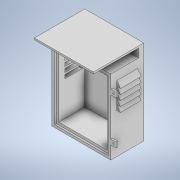
# Autodesk Inventor part: Part6
Saved by Autodesk Inventor 2022.6 (Build 266554010, 554A)
## iProperties
Created: 2025-03-19
Part Number: Part6
Material: Generic
Document SubType Name: Modeling
Designer: khinm
Density: 1 g/cm^3
Appearance: Default
Author: khinm
Autodesk Inventor part; units mm, degrees
sketch "Sketch2" plane through (0, 0, 0) normal (1, 0, 0) x (0, 1, 0)
  line L0 (215, 47.5) -> (0, 47.5)
  line L1 (0, 47.5) -> (0, -47.5)
  line L2 (0, -47.5) -> (215, -47.5)
  line L3 (215, -47.5) -> (215, 47.5)
  point P0 (0, 0)
  point P1 (0, 0)
  dimension "d0" = 95
  dimension "d1" = 215
  constraints: 8 end point, 2 parallel, 1 coincident, 1 horizontal, 1 midpoint, 1 perpendicular
  measures "d0" distance of L2.end L0.start
  measures "d1" distance from line of L1.end L3
extrude "Extrusion1" add sketch "Sketch2" along normal mid plane 170
sketch "Sketch3" plane through (-85, 0, 47.5) normal (0, 0, 1) x (1, 0, 0)
  line L0 (15, 200) -> (155, 200)
  line L1 (155, 200) -> (155, 15)
  line L2 (155, 15) -> (15, 15)
  line L3 (15, 15) -> (15, 200)
  line L4 (170, 0) -> (0, 0) projected
  line L5 (0, 215) -> (170, 215) projected
  line L6 (0, 0) -> (0, 215) projected
  line L7 (170, 215) -> (170, 0) projected
  point P0 (85, 0)
  point P1 (85, 0)
  point P2 (85, 15)
  dimension "d4" = 15
  dimension "d5" = 15
  dimension "d6" = 15
  dimension "d7" = 15
  constraints: 8 end point, 2 midpoint, 2 parallel, 1 horizontal, 1 perpendicular, 1 vertical alignment
  measures "d4" distance between parallel lines of L5 L0
  measures "d5" distance between parallel lines of L4 L2
  measures "d6" distance between parallel lines of L6 L3
  measures "d7" distance between parallel lines of L1 L7
extrude "Extrusion2" cut sketch "Sketch3" against normal blind 80 contours L0 L1 L2 L3
ref_plane "Work Plane1" through (0, 0, 0) normal (1, 0, 0) x (0, 1, 0)
sketch "Sketch4" plane through (0, 0, 0) normal (1, 0, 0) x (0, 1, 0)
  line L0 (200, 47.5) -> (200, -32.5) projected
  line L1 (15, 47.5) -> (200, 47.5) projected
  line L2 (200, 47.5) -> (207.5, 47.5)
  line L3 (207.5, 47.5) -> (207.5, 42.5)
  line L4 (207.5, 42.5) -> (200, 42.5)
  line L5 (200, 42.5) -> (200, 47.5)
  point P0 (0, 0)
  point P1 (200, 45)
  point P2 (207.5, 45)
  point P3 (203.75, 42.5)
  point P4 (203.75, 47.5)
  dimension "d12" = 7.5
  dimension "d13" = 5
  constraints: 8 end point, 4 midpoint, 2 parallel, 1 horizontal, 1 perpendicular
  measures "d12" distance of point (200, 45) point (207.5, 45)
  measures "d13" distance of point (203.75, 42.5) point (203.75, 47.5)
sketch3d "3D Sketch1"
  line L0 (-70, 200, 47.5) -> (-70, 15, 47.5)
  line L1 (-70, 15, 47.5) -> (70, 15, 47.5)
  line L2 (70, 15, 47.5) -> (70, 200, 47.5)
  line L3 (70, 200, 47.5) -> (-70, 200, 47.5)
sweep "Sweep1" cut profiles "Sketch4" path "3D Sketch1"
ref_plane "Work Plane2" through (0, 0, 0) normal (0, 0, 1) x (1, 0, 0)
sketch "Sketch6" plane through (0, 0, 0) normal (0, 0, 1) x (1, 0, 0)
  line L0 (85, 0) -> (85, 215) projected
  line L1 (85, 190) -> (85, 175)
  line L2 (85, 175) -> (95, 175)
  line L3 (95, 175) -> (85, 190)
  point P0 (0, 0)
  dimension "d17" = 25
  dimension "d18" = 15
  dimension "d19" = 10
  dimension "d23" = 56.31
  constraints: 6 end point, 2 point on line, 1 horizontal
  measures "d17" distance of L1.start L0.end
  measures "d18" distance of L1.end L1.start
  measures "d19" distance of L1.end L2.end
  measures "d23" angle of L3 L2
extrude "Extrusion3" add sketch "Sketch6" along normal mid plane 60
sketch "Sketch7" plane through (0, 0, 0) normal (0, 0, 1) x (1, 0, 0)
  line L0 (70, 200) -> (70, 15) projected
  line L1 (70, 175) -> (91.6667, 175)
  line L2 (85, 0) -> (85, 215) projected
  line L3 (91.6667, 175) -> (85, 185)
  line L4 (85, 190) -> (95, 175) projected
  line L5 (85, 185) -> (70, 185)
  line L6 (70, 185) -> (70, 175)
  point P0 (0, 0)
  dimension "d22" = 10
  constraints: 8 end point, 2 parallel, 2 point on line, 1 collinear, 1 horizontal alignment, 1 perpendicular, 1 vertical alignment
  measures "d22" distance between parallel lines of L5 L1
extrude "Extrusion4" cut sketch "Sketch7" along normal mid plane 50
pattern_linear "Rectangular Pattern1" count 5 spacing 15 along (0, -1, 0) of "Extrusion3", "Extrusion4"
mirror "Mirror1" about plane through (0, 0, 0) normal (1, 0, 0) of "Extrusion3", "Extrusion4", "Rectangular Pattern1"
ref_plane "Work Plane4" through (0, 0, 47.5) normal (0, 0, 1) x (1, 0, 0)
sketch "Sketch8" plane through (0, 0, 47.5) normal (0, 0, 1) x (1, 0, 0)
  line L0 (85, 215) -> (85, 0) projected
  line L1 (85, 0) -> (85, 215) projected
  line L2 (85, 162.5) -> (100, 162.5)
  line L3 (100, 162.5) -> (100, 177.5)
  line L4 (100, 177.5) -> (85, 177.5)
  line L5 (85, 177.5) -> (85, 162.5)
  point P0 (0, 0)
  dimension "d31" = 52.5
  dimension "d32" = 15
  dimension "d33" = 15
  constraints: 8 end point, 2 parallel, 1 horizontal, 1 perpendicular, 1 point on line
  measures "d31" distance of L2.start L0.start
  measures "d32" distance of L2.end L3.end
  measures "d33" distance of L2.end L2.start
extrude "Extrusion5" add sketch "Sketch8" against normal blind 5
ref_plane "Work Plane5" through (0, 107.5, 0) normal (0, 1, 0) x (-1, 0, 0)
sketch "Sketch9" plane through (-85, 0, 47.5) normal (0, 0, 1) x (1, 0, 0)
  line L0 (185, 177.5) -> (170, 177.5) projected
  line L1 (185, 162.5) -> (185, 177.5) projected
  point P0 (85, 0)
  point P1 (177.5, 170)
  point P2 (177.5, 177.5)
  dimension "d37" = 7.5
  dimension "d38" = 7.5
  constraints: 1 midpoint
  measures "d37" distance of point (177.5, 177.5) point (177.5, 170)
  measures "d38" distance from line of L1 point (177.5, 170)
hole "Hole1" at (92.5, 170, 47.5) direction (0, 0, -1) diameter 4.134 depth 5 tip angle 118
mirror "Mirror3" about plane through (0, 107.5, 0) normal (0, 1, 0) of "Extrusion5", "Hole1"
sketch "Sketch10" plane through (-85, 215, 47.5) normal (0, 1, 0) x (1, 0, 0)
  line L0 (0, 0) -> (170, 0) projected
  line L1 (170, 95) -> (170, 0) projected
  line L2 (0, 95) -> (170, 95) projected
  line L3 (0, 0) -> (0, 95) projected
  line L4 (0, 95) -> (170, 95)
  line L5 (170, 95) -> (170, 80)
  line L6 (170, 80) -> (0, 80)
  line L7 (0, 80) -> (0, 95)
  point P0 (85, 47.5)
  dimension "d46" = 15
  dimension "d47" = 170
  constraints: 8 end point, 2 parallel, 1 horizontal, 1 perpendicular
  measures "d46" distance of L5.end L4.end
  measures "d47" distance of L2.start L4.end
extrude "Extrusion6" add sketch "Sketch10" along normal blind 30 contours L3 L2 L1 L6
sketch "Sketch12" plane through (-85, 215, -32.5) normal (0, 0, 1) x (1, 0, 0)
  line L0 (0, 30) -> (170, 30) projected
  line L1 (0, 30) -> (170, 30)
  line L2 (170, 30) -> (170, 25)
  line L3 (170, 25) -> (0, 25)
  line L4 (0, 25) -> (0, 30)
  point P0 (85, -215)
  point P1 (170, 27.5)
  point P2 (0, 27.5)
  dimension "d52" = 5
  dimension "d53" = 170
  constraints: 8 end point, 2 midpoint, 2 parallel, 1 horizontal, 1 perpendicular
  measures "d52" distance of L2.end L1.end
  measures "d53" distance of point (170, 27.5) point (0, 27.5)
extrude "Extrusion7" add sketch "Sketch12" along normal blind 130
body "Solid1"
